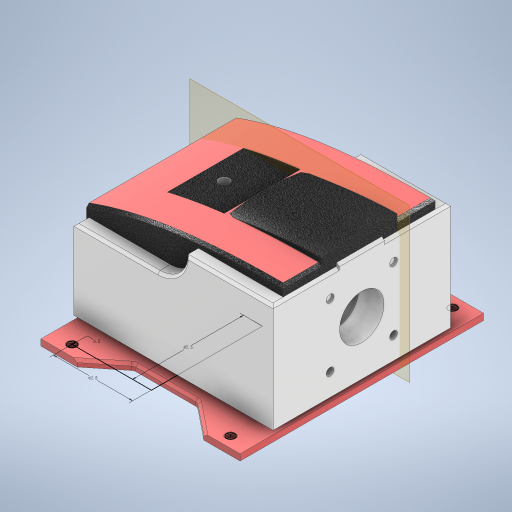
# Autodesk Inventor part: laser_base
Saved by Autodesk Inventor 2023.5 (Build 275446000, 446)
## iProperties
Created: 2025-03-29
Part Number: laser_base
Material: 常规
Document SubType Name: Modeling
Designer: jiaxue
Density: 1 g/cm^3
Appearance: 平滑 - 白色
Author: jiaxue
Autodesk Inventor part; units mm, degrees
note: some values were not read from the file. Chosen so that the rebuilt part matches the saved one: second side of "拉伸8".
ref_plane "YZ Plane" through (0, 0, 0) normal (1, 0, 0) x (0, 1, 0)
ref_plane "XZ Plane" through (0, 0, 0) normal (0, 1, 0) x (-1, 0, 0)
ref_plane "XY Plane" through (0, 0, 0) normal (0, 0, 1) x (1, 0, 0)
sketch "草图1" plane through (0, 0, 0) normal (0, 1, 0) x (-1, 0, 0)
  line L0 (-78.5, 96) -> (78.5, 96)
  line L1 (78.5, 96) -> (78.5, -96)
  line L2 (78.5, -96) -> (-78.5, -96)
  line L3 (-78.5, -96) -> (-78.5, 96)
  line L4 (-78.5, 96) -> (78.5, -96) construction
  line L5 (78.5, 96) -> (-78.5, -96) construction
  point P0 (0, 0)
  dimension "d0" = 157
  dimension "d1" = 192
  constraints: 12 end point, 2 midpoint, 2 parallel, 1 horizontal, 1 perpendicular
  measures "d0" distance of L1.end L2.end
  measures "d1" distance of L1.end L0.end
extrude "拉伸1" add sketch "草图1" along normal blind 5
sketch "草图2" plane through (0, 5, 0) normal (0, 1, 0) x (1, 0, 0)
  line L0 (0, 0) -> (0, -87.5)
  line L1 (0, -87.5) -> (-62.5, -87.5)
  line L2 (0, 0) -> (-7.1, 0)
  circle A0 centre (-62.5, -87.5) radius 3.25
  circle A1 centre (-62.5, 87.5) radius 3.25
  circle A2 centre (62.5, -87.5) radius 3.25
  circle A3 centre (62.5, 87.5) radius 3.25
  dimension "d4" = 87.5
  dimension "d6" = 62.5
  dimension "d86" = 6.5
  constraints: 9 symmetric about line, 6 end point, 4 centre point, 4 coincident, 2 horizontal, 1 vertical, 3 other
  measures "d4" distance of L0.start L0.end
  measures "d6" distance of L0.end L1.end
  measures "d86" diameter of A0
sketch "草图3" plane through (0, 5, 0) normal (0, 1, 0) x (1, 0, 0)
  circle A0 centre (0, 0) radius 30
  dimension "d14" = 60
  constraints: 1 centre point, 1 coincident
  measures "d14" diameter of A0
extrude "拉伸2" add sketch "草图3" along normal blind 3
sketch "草图4" plane through (0, 8, 0) normal (0, 1, 0) x (1, 0, 0)
  line L0 (-78.5, 96) -> (-78.5, -96) projected
  line L1 (78.5, -70) -> (-78.5, -70)
  line L2 (-78.5, -70) -> (-78.5, 70)
  line L3 (-78.5, 70) -> (78.5, 70)
  line L4 (78.5, 70) -> (78.5, -70)
  line L5 (78.5, -70) -> (-78.5, 70) construction
  line L6 (-78.5, -70) -> (78.5, 70) construction
  point P0 (0, 0)
  dimension "d17" = 140
  constraints: 12 end point, 2 midpoint, 2 parallel, 1 horizontal, 1 perpendicular, 1 point on line
  measures "d17" distance between parallel lines of L3 L1
extrude "拉伸3" add sketch "草图4" along normal blind 85
sketch "草图5" plane through (78.5, 8, 70) normal (1, 0, 0) x (0, 0, -1)
  line L0 (140, 85) -> (0, 85) projected
  line L1 (70, 85) -> (70, 0)
  line L2 (100, 0) -> (40, 0) projected
  line L3 (0, 0) -> (0, 85) projected
  line L4 (0, 42.5) -> (140, 42.5)
  line L5 (140, 0) -> (140, 85) projected
  circle A0 centre (70, 42.5) radius 17.5
  point P0 (70, -8)
  dimension "d20" = 35
  constraints: 5 midpoint, 4 end point, 1 centre point
  measures "d20" diameter of A0
extrude "拉伸4" cut sketch "草图5" against normal blind 20 contours A0 L4 L1 | L1 L4 A0 | A0 L1 L4 | L1 A0 L4
sketch "草图6" plane through (78.5, 8, 70) normal (1, 0, 0) x (0, 0, -1)
  line L0 (45, 17.5) -> (95, 17.5)
  line L1 (95, 17.5) -> (95, 67.5)
  line L2 (95, 67.5) -> (45, 67.5)
  line L3 (45, 67.5) -> (45, 17.5)
  circle A0 centre (70, 42.5) radius 17.5 projected
  line L4 (45, 17.5) -> (95, 67.5) construction
  line L5 (95, 17.5) -> (45, 67.5) construction
  point P0 (70, -8)
  dimension "d23" = 50
  dimension "d24" = 50
  constraints: 12 end point, 2 midpoint, 2 parallel, 1 horizontal, 1 perpendicular
  measures "d23" distance of L2.end L1.end
  measures "d24" distance of L1.end L0.end
hole "孔2" at (78.5, 75.5, 25) at (78.5, 25.5, 25) at (78.5, 25.5, -25) at (78.5, 75.5, -25) direction (-1, 0, 0) diameter 6 depth 10 tip angle 118
sketch "草图7" plane through (-78.5, 8, 70) normal (0, 0, 1) x (1, 0, 0)
  line L0 (157, 85) -> (0, 85) projected
  line L1 (157, 85) -> (157, 62.8383)
  line L2 (157, 0) -> (157, 85) projected
  line L3 (66.0882, 62.8383) -> (0, 62.8383)
  line L4 (0, 0) -> (0, 85) projected
  arc A0 (66.0882, 62.8383) -> (88.2499, 85) centre (66.0882, 85) ccw
  line L5 (0, 62.8383) -> (0, 85)
  point P0 (78.5, -8)
  constraints: 6 end point, 2 point on circle, 2 point on line, 1 centre point, 1 horizontal, 1 tangent, 1 vertical
extrude "拉伸5" cut sketch "草图7" against normal blind 70
mirror "镜像1" about plane through (0, 0, 0) normal (0, 0, 1) of "拉伸5"
sketch "草图9" plane through (0, 0, 0) normal (0, 0, 1) x (1, 0, 0)
  line L0 (-78.5, 70.8383) -> (76.5, 70.8383)
  line L1 (-12.4118, 70.8383) -> (-78.5, 70.8383) projected
  line L2 (76.5, 70.8383) -> (76.5, 100.8383)
  line L3 (-78.5, 70.8383) -> (-78.5, 78.8383)
  line L4 (76.5, 100.8383) -> (6.0658, 100.8383) construction
  line L5 (9.7499, 93) -> (78.5, 93) projected
  line L6 (6.0658, 100.8383) -> (-39.9065, 93) construction
  line L7 (-39.9065, 93) -> (-78.5, 78.8383) construction
  spline S0 degree 3 poles (76.5, 100.8383) (6.0658, 100.8383) (-39.9065, 93) (-78.5, 78.8383) knots 1 1 1 1 2 2 2 2
  point P0 (0, 0)
  dimension "d44" = 155
  dimension "d45" = 30
  dimension "d46" = 8
  constraints: 6 end point, 1 collinear, 1 parallel, 1 perpendicular, 1 vertical, 3 other
  measures "d44" distance of L0.start L0.end
  measures "d45" distance of L0.end L2.end
  measures "d46" distance of L0.start L3.end
extrude "拉伸7" add sketch "草图9" along normal mid plane 120
chamfer "倒角3" distance 2 angle 45 13 edges at (78.5, 93, 0) (44.1249, 93, -70) (3.2589, 77.3293, -70) (-45.4559, 70.8383, -70) (-78.5, 70.8383, -65) (-78.5, 70.8383, 65) (-45.4559, 70.8383, 70) (3.2589, 77.3293, 70) (44.1249, 93, 70) (-12.9403, 95.1489, -60) (76.5, 100.8383, -30) (76.5, 100.8383, 30) (-12.9403, 95.1489, 60)
sketch "草图10" plane through (0, 0, 0) normal (1, 0, 0) x (0, 1, 0)
  line L0 (97, -30) -> (89, -30)
  line L1 (89, -30) -> (89, 30)
  line L2 (89, 30) -> (97, 30)
  line L3 (97, 30) -> (97, -30)
  line L4 (93, -60) -> (93, 60) projected
  line L5 (97, -30) -> (89, 30) construction
  line L6 (89, -30) -> (97, 30) construction
  point P0 (0, 0)
  point P1 (93, 0)
  dimension "d52" = 8
  dimension "d53" = 60
  constraints: 12 end point, 3 midpoint, 2 parallel, 1 horizontal, 1 perpendicular
  measures "d52" distance of L1.end L2.end
  measures "d53" distance of L0.end L1.end
extrude "拉伸8" cut sketch "草图10" against normal blind 61.75
sketch "草图11" plane through (0, 89, 30) normal (0, 1, 0) x (1, 0, 0)
  circle A0 centre (0, 30) radius 30 projected
  circle A1 centre (-30, 30) radius 5
  dimension "d58" = 10
  constraints: 1 centre point, 1 horizontal alignment, 1 other
  measures "d58" diameter of A1
hole "孔3" at (-30, 89, 0) direction (0, -1, 0) diameter 8.376 depth 10 tip angle 118
sketch "草图12" plane through (78.5, 8, 70) normal (1, 0, 0) x (0, 0, -1)
  line L0 (52.165, 78.4805) -> (87.835, 78.4805)
  line L1 (87.835, 78.4805) -> (87.835, 87.5195)
  line L2 (87.835, 87.5195) -> (52.165, 87.5195)
  line L3 (52.165, 87.5195) -> (52.165, 78.4805)
  line L4 (0, 83) -> (140, 83) projected
  line L5 (52.165, 78.4805) -> (87.835, 87.5195) construction
  line L6 (87.835, 78.4805) -> (52.165, 87.5195) construction
  point P0 (70, -8)
  point P1 (70, 83)
  constraints: 12 end point, 3 midpoint, 2 parallel, 1 horizontal, 1 perpendicular
extrude "拉伸9" add sketch "草图12" against normal blind 27
chamfer "倒角4" distance 2 angle 45 1 edges at (78.5, 95.5195, 0)
sketch "草图13" plane through (76.5, 93, -60) normal (1, 0, 0) x (0, 0, -1)
  line L0 (-90, 3.8699) -> (-90, -4) projected
  line L1 (-90, 3.8699) -> (-30, 3.8699)
  line L2 (-30, 3.8699) -> (-30, 11.8699)
  line L3 (-90, 3.8699) -> (-90, 11.8699)
  line L4 (-90, 11.8699) -> (-60, 16.8318) construction
  line L5 (-60, 16.8318) -> (-30, 11.8699) construction
  spline S0 degree 2 poles (-90, 11.8699) (-60, 16.8318) (-30, 11.8699) knots 1 1 1 2 2 2
  point P0 (-60, -93)
  dimension "d71" = 60
  dimension "d72" = 8
  dimension "d73" = 8
  constraints: 6 end point, 1 horizontal, 1 perpendicular, 1 vertical, 3 other
  measures "d71" distance of L0.start L1.end
  measures "d72" distance of L1.end L2.end
  measures "d73" distance of L0.start L3.end
ref_plane "工作平面1" through (76.5, 96.8699, -30) normal (0, 0, 1) x (0, 1, 0)
sketch "草图14" plane through (76.5, 96.8699, -30) normal (0, 0, 1) x (0, 1, 0)
  line L0 (8, 0) -> (8, 27.6413) construction
  line L1 (8, 27.6413) -> (0, 74) construction
  spline S0 degree 2 poles (8, 0) (8, 27.6413) (0, 74) knots 1 1 1 2 2 2
  point P0 (-96.8699, 76.5)
  constraints: 1 vertical, 3 other
sweep "扫掠1" add profiles "草图13" path "草图14"
sketch "草图16" plane through (0, 0, 0) normal (0, -1, 0) x (1, 0, 0)
  line L0 (-25, 58.5392) -> (-3.1741, 58.5392)
  line L1 (-50, 108.5) -> (-50, 96)
  line L2 (-78.5, 96) -> (78.5, 96) projected
  line L3 (-58.4797, 49.2162) -> (58.4797, 142.7838) construction
  line L4 (40.4778, 63.6177) -> (-40.4778, 128.3823) construction
  line L5 (25, 96) -> (25, 76)
  line L6 (25, 76) -> (-25, 76)
  line L7 (-25, 76) -> (-25, 96)
  line L8 (-25, 116) -> (25, 76) construction
  line L9 (25, 116) -> (-25, 76) construction
  line L10 (50, 96) -> (25, 76)
  line L11 (-50, 96) -> (-25, 76)
  line L12 (50, 96) -> (-50, 96)
  point P0 (0, 0)
  point P1 (0, 96)
  dimension "d77" = 100
  dimension "d78" = 50
  dimension "d79" = 20
  constraints: 24 end point, 9 point on line, 5 midpoint, 1 collinear, 1 horizontal, 1 parallel
  measures "d77" distance of L4.end L3.end
  measures "d78" distance of L5.end L6.end
  measures "d79" distance between parallel lines of L12 L6
extrude "拉伸10" cut sketch "草图16" against normal up to surface (5 mm away)
mirror "镜像2" about plane through (0, 0, 0) normal (0, 0, 1) of "拉伸10"
fillet "圆角1" radius 4 4 edges at (-25, 2.5, 76) (25, 2.5, 76) (-25, 2.5, -76) (25, 2.5, -76)
chamfer "倒角5" distance 2 angle 45 10 edges at (0, 5, -76) (-24.9209, 5, -76.2255) (-38.0478, 5, -86.4383) (24.9209, 5, -76.2255) (38.0478, 5, -86.4383) (0, 5, 76) (24.9209, 5, 76.2255) (38.0478, 5, 86.4383) (-24.9209, 5, 76.2255) (-38.0478, 5, 86.4383)
extrude "拉伸11" cut sketch "草图2" against normal blind 10
thread "螺纹1"
thread "螺纹2"
thread "螺纹3"
thread "螺纹4"
chamfer "倒角6" distance 0.5 angle 45 4 edges at (59.25, 5, -87.5) (59.25, 5, 87.5) (-65.75, 5, -87.5) (-65.75, 5, 87.5)
